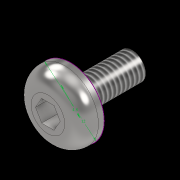
# Autodesk Inventor part: SkaterInsertScrew
Saved by Autodesk Inventor 2022.2 (Build 262287010, 287A)
## iProperties
Created: 2022-06-03
Part Number: SkaterInsertScrew
Material: Stainless Steel
Document SubType Name: Modeling
Designer: Árni Þór Þorgeirsson
Density: 8 g/cm^3
Appearance: Semi-Polished
Author: Árni Þór Þorgeirsson
Autodesk Inventor part; units mm, degrees
ref_plane "YZ Plane" through (0, 0, 0) normal (1, 0, 0) x (0, 1, 0)
ref_plane "XZ Plane" through (0, 0, 0) normal (0, 1, 0) x (-1, 0, 0)
ref_plane "XY Plane" through (0, 0, 0) normal (0, 0, 1) x (1, 0, 0)
sketch "Sketch1" plane through (0, 0, 0) normal (0, 0, 1) x (1, 0, 0)
  circle A0 centre (0, 0) radius 2.4
  circle A1 centre (0, 0) radius 6
  dimension "d0" = 4.8
  dimension "d1" = 12
  constraints: 2 centre point, 2 coincident
  measures "d0" diameter of A0
  measures "d1" diameter of A1
extrude "Extrusion1" add sketch "Sketch1" along normal blind 4 contours A0 | A1
extrude "Extrusion2" add sketch "Sketch1" against normal blind 11 contours A0
fillet "Fillet1" radius 1 1 edges at (-2.4, 0, 0)
fillet "Fillet2" radius 3 1 edges at (-6, 0, 4)
sketch "Sketch2" plane through (0, 0, 4) normal (0, 0, 1) x (1, 0, 0)
  line L0 (2.2, 0) -> (1.1, -1.9053)
  line L1 (1.1, -1.9053) -> (-1.1, -1.9053)
  line L2 (-1.1, -1.9053) -> (-2.2, 0)
  line L3 (-2.2, 0) -> (-1.1, 1.9053)
  line L4 (-1.1, 1.9053) -> (1.1, 1.9053)
  line L5 (1.1, 1.9053) -> (2.2, 0)
  point P0 (0, 0)
  point P1 (0, 0)
  dimension "d8" = 4.4
  constraints: 12 end point, 1 coincident, 13 other
  measures "d8" distance of L0.start L2.end
extrude "Extrusion3" cut sketch "Sketch2" against normal blind 3
thread "Thread1" size "M5x0.8" class "6g" standard "ANSI Metric M Profile" full length
body "Solid1"
